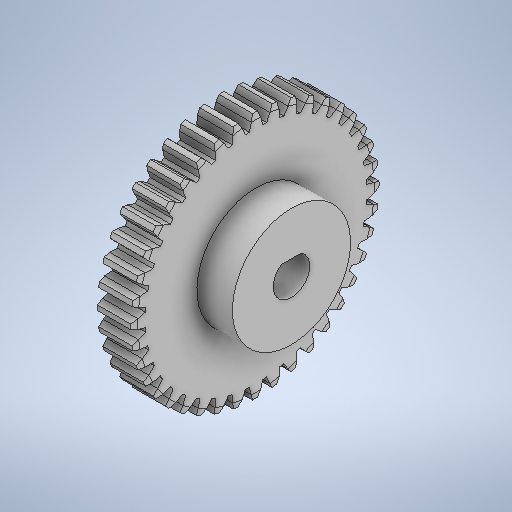
# Autodesk Inventor part: HPC - G1-40 (C)
Saved by Autodesk Inventor 2025.2 (Build 292293000, 293)
## iProperties
Category: PARTsolutions
Company: HPC
Created: 2025-05-10
Part Number: HPC - G1-40 (C)
Material: Generic
Catalog Web Link: www.cadenas.de
Description: G/PG 1-Spur gear - Steel 20NCD2 - Module 1.0
Vendor: HPC
Document SubType Name: Modeling
Designer: psAdmin
Manufacturer: HPC
Mass: 98 g
Surface Area: 56.4798 cm^2
Volume: 12.7412 cm^3
Density: 1 g/cm^3
Appearance: PSOLRGB-175-175-175
PSOL_IDENT_0: {$CADENAS_DATA/23d-libs/hpc/v4/spur_gear/100/g1.prj},171 {VTYP=3D},{NB=HPC - G1-40 (C)},{LINA=HPC -
PSOL_IDENT_1: G1-40},{NN=G/PG 1},{DATE=17.02.2022 08:08:10},{GEOMDATE=24.09.2019 07:57:00},{VERSION=},{LINEID=1130
PSOL_IDENT_2: },{WBVAR=DET},{WBNUMERIC=}  {NB=hpc_G1-40_C},{LINA=HPC - G1-40},{KT=DUMMY},{REF=G1-40},{DET=C},{TYP=
PSOL_IDENT_3: G},{MOD=1.0},{Z=40},{P=40.00},{D=42.00},{M=20},{MX=20.000},{A=8},{MAS=0.098},{INFO=INFO},{MODULE=1.0
PSOL_IDENT_4: 00},{X=37.5},{HIDDENLINE=V}
NB: HPC - G1-40 (C)
NN: G/PG 1
NT: Spur gear - Steel 20NCD2 - Module 1.0
NBSYN: HPC - $REF. ($DET.)
LINA: HPC - G1-40
CATALOG: HPC
REF: G1-40
DET: Full
TYP: G
MOD: 1.0
Z: 40
P: 40
D: 42
M: 20
A: 8
MAS: 0.098
INFO: INFO
SUPPLIER: HPC
ARTICLENO: HPC - G1-40 (C)
BOMINFO: HPC - G1-40
CREATOR: CADENAS GmbH
Title: HPC - G1-40
Author: Cadenas PARTsolutions
Comments: Spur gear - Steel 20NCD2 - Module 1.0
Autodesk Inventor part; units mm, degrees
ref_plane "YZ Plane" through (0, 0, 0) normal (1, 0, 0) x (0, 1, 0)
ref_plane "XZ Plane" through (0, 0, 0) normal (0, 1, 0) x (-1, 0, 0)
ref_plane "XY Plane" through (0, 0, 0) normal (0, 0, 1) x (1, 0, 0)
sketch "Esquisse_1" plane through (0, 0, 0) normal (0, 0, 1) x (1, 0, 0)
  line L0 (8, 0) -> (0, 0)
  line L1 (0, 20) -> (0, 0)
  line L2 (6, 20) -> (5.8237, 21)
  line L3 (5.8237, 21) -> (0.1763, 21)
  line L4 (0.1763, 21) -> (0, 20)
  line L5 (12, 0) -> (12, 10)
  line L6 (12, 10) -> (6, 10)
  line L7 (0, 0) -> (12, 0)
  line L8 (6, 10) -> (6, 20)
  dimension "d12" = 20
  dimension "d13" = 42
  dimension "d18" = 20
  dimension "d20" = 1
  dimension "d21" = 170
  dimension "d22" = 1
  dimension "d23" = 6
  dimension "d24" = 12
  constraints: 18 end point, 4 parallel, 2 horizontal, 1 vertical, 2 other
  measures "d12" diameter of L6 L0
  measures "d13" diameter of L3 L0
  measures "d18" angle of L2 L4
  measures "d20" vertical distance of L2.end L2.start
  measures "d21" angle of L4 L1
  measures "d22" vertical distance of L1.start L3.end
  measures "d23" distance between parallel lines of L8 L1
  measures "d24" distance between parallel lines of L5 L1
revolve "Revolution1" add sketch "Esquisse_1" angle 360 about axis through (8, 0, 0) along (1, 0, 0)
sketch "Esquisse_2" plane through (0, 0, 0) normal (1, 0, 0) x (0, 1, 0)
  line L0 (-23, 23) -> (-23, -23)
  line L1 (-23, -23) -> (23, -23)
  line L2 (23, -23) -> (23, 23)
  line L3 (23, 23) -> (-23, 23)
  arc A0 (0.344, 21.1972) -> (-0.344, 21.1972) centre (0, 0) ccw
  line L4 (-0.344, 21.1972) -> (-0.7854, 19.9846)
  line L5 (-0.7854, 19.9846) -> (-1.1253, 18.7162)
  arc A1 (-1.1253, 18.7162) -> (-1.8165, 18.6618) centre (0, 0) ccw
  line L6 (-1.8165, 18.6618) -> (-2.3505, 19.8614)
  line L7 (-2.3505, 19.8614) -> (-2.9762, 20.9901)
  arc A2 (-2.9762, 20.9901) -> (-3.6558, 20.8824) centre (0, 0) ccw
  line L8 (-3.6558, 20.8824) -> (-3.902, 19.6157)
  line L9 (-3.902, 19.6157) -> (-4.0393, 18.3097)
  arc A3 (-4.0393, 18.3097) -> (-4.7134, 18.1479) centre (0, 0) ccw
  line L10 (-4.7134, 18.1479) -> (-5.4286, 19.2492)
  line L11 (-5.4286, 19.2492) -> (-6.2231, 20.2661)
  arc A4 (-6.2231, 20.2661) -> (-6.8775, 20.0534) centre (0, 0) ccw
  line L12 (-6.8775, 20.0534) -> (-6.9225, 18.7638)
  line L13 (-6.9225, 18.7638) -> (-6.8538, 17.4524)
  arc A5 (-6.8538, 17.4524) -> (-7.4944, 17.1871) centre (0, 0) ccw
  line L14 (-7.4944, 17.1871) -> (-8.373, 18.1629)
  line L15 (-8.373, 18.1629) -> (-9.3168, 19.043)
  arc A6 (-9.3168, 19.043) -> (-9.9299, 18.7307) centre (0, 0) ccw
  line L16 (-9.9299, 18.7307) -> (-9.7726, 17.4498)
  line L17 (-9.7726, 17.4498) -> (-9.4996, 16.1654)
  arc A7 (-9.4996, 16.1654) -> (-10.0908, 15.8031) centre (0, 0) ccw
  line L18 (-10.0908, 15.8031) -> (-11.1112, 16.6295)
  line L19 (-11.1112, 16.6295) -> (-12.1811, 17.3511)
  arc A8 (-12.1811, 17.3511) -> (-12.7377, 16.9467) centre (0, 0) ccw
  line L20 (-12.7377, 16.9467) -> (-12.382, 15.7062)
  line L21 (-12.382, 15.7062) -> (-11.9115, 14.4803)
  arc A9 (-11.9115, 14.4803) -> (-12.4387, 14.03) centre (0, 0) ccw
  line L22 (-12.4387, 14.03) -> (-13.5759, 14.6866)
  line L23 (-13.5759, 14.6866) -> (-14.7454, 15.232)
  arc A10 (-14.7454, 15.232) -> (-15.232, 14.7454) centre (0, 0) ccw
  line L24 (-15.232, 14.7454) -> (-14.6866, 13.5759)
  line L25 (-14.6866, 13.5759) -> (-14.03, 12.4387)
  arc A11 (-14.03, 12.4387) -> (-14.4803, 11.9115) centre (0, 0) ccw
  line L26 (-14.4803, 11.9115) -> (-15.7062, 12.382)
  line L27 (-15.7062, 12.382) -> (-16.9467, 12.7377)
  arc A12 (-16.9467, 12.7377) -> (-17.3511, 12.1811) centre (0, 0) ccw
  line L28 (-17.3511, 12.1811) -> (-16.6295, 11.1112)
  line L29 (-16.6295, 11.1112) -> (-15.8031, 10.0908)
  arc A13 (-15.8031, 10.0908) -> (-16.1654, 9.4996) centre (0, 0) ccw
  line L30 (-16.1654, 9.4996) -> (-17.4498, 9.7726)
  line L31 (-17.4498, 9.7726) -> (-18.7307, 9.9299)
  arc A14 (-18.7307, 9.9299) -> (-19.043, 9.3168) centre (0, 0) ccw
  line L32 (-19.043, 9.3168) -> (-18.1629, 8.373)
  line L33 (-18.1629, 8.373) -> (-17.1871, 7.4944)
  arc A15 (-17.1871, 7.4944) -> (-17.4524, 6.8538) centre (0, 0) ccw
  line L34 (-17.4524, 6.8538) -> (-18.7638, 6.9225)
  line L35 (-18.7638, 6.9225) -> (-20.0534, 6.8775)
  arc A16 (-20.0534, 6.8775) -> (-20.2661, 6.2231) centre (0, 0) ccw
  line L36 (-20.2661, 6.2231) -> (-19.2492, 5.4286)
  line L37 (-19.2492, 5.4286) -> (-18.1479, 4.7134)
  arc A17 (-18.1479, 4.7134) -> (-18.3097, 4.0393) centre (0, 0) ccw
  line L38 (-18.3097, 4.0393) -> (-19.6157, 3.902)
  line L39 (-19.6157, 3.902) -> (-20.8824, 3.6558)
  arc A18 (-20.8824, 3.6558) -> (-20.9901, 2.9762) centre (0, 0) ccw
  line L40 (-20.9901, 2.9762) -> (-19.8614, 2.3505)
  line L41 (-19.8614, 2.3505) -> (-18.6618, 1.8165)
  arc A19 (-18.6618, 1.8165) -> (-18.7162, 1.1253) centre (0, 0) ccw
  line L42 (-18.7162, 1.1253) -> (-19.9846, 0.7854)
  line L43 (-19.9846, 0.7854) -> (-21.1972, 0.344)
  arc A20 (-21.1972, 0.344) -> (-21.1972, -0.344) centre (0, 0) ccw
  line L44 (-21.1972, -0.344) -> (-19.9846, -0.7854)
  line L45 (-19.9846, -0.7854) -> (-18.7162, -1.1253)
  arc A21 (-18.7162, -1.1253) -> (-18.6618, -1.8165) centre (0, 0) ccw
  line L46 (-18.6618, -1.8165) -> (-19.8614, -2.3505)
  line L47 (-19.8614, -2.3505) -> (-20.9901, -2.9762)
  arc A22 (-20.9901, -2.9762) -> (-20.8824, -3.6558) centre (0, 0) ccw
  line L48 (-20.8824, -3.6558) -> (-19.6157, -3.902)
  line L49 (-19.6157, -3.902) -> (-18.3097, -4.0393)
  arc A23 (-18.3097, -4.0393) -> (-18.1479, -4.7134) centre (0, 0) ccw
  line L50 (-18.1479, -4.7134) -> (-19.2492, -5.4286)
  line L51 (-19.2492, -5.4286) -> (-20.2661, -6.2231)
  arc A24 (-20.2661, -6.2231) -> (-20.0534, -6.8775) centre (0, 0) ccw
  line L52 (-20.0534, -6.8775) -> (-18.7638, -6.9225)
  line L53 (-18.7638, -6.9225) -> (-17.4524, -6.8538)
  arc A25 (-17.4524, -6.8538) -> (-17.1871, -7.4944) centre (0, 0) ccw
  line L54 (-17.1871, -7.4944) -> (-18.1629, -8.373)
  line L55 (-18.1629, -8.373) -> (-19.043, -9.3168)
  arc A26 (-19.043, -9.3168) -> (-18.7307, -9.9299) centre (0, 0) ccw
  line L56 (-18.7307, -9.9299) -> (-17.4498, -9.7726)
  line L57 (-17.4498, -9.7726) -> (-16.1654, -9.4996)
  arc A27 (-16.1654, -9.4996) -> (-15.8031, -10.0908) centre (0, 0) ccw
  line L58 (-15.8031, -10.0908) -> (-16.6295, -11.1112)
  line L59 (-16.6295, -11.1112) -> (-17.3511, -12.1811)
  arc A28 (-17.3511, -12.1811) -> (-16.9467, -12.7377) centre (0, 0) ccw
  line L60 (-16.9467, -12.7377) -> (-15.7062, -12.382)
  line L61 (-15.7062, -12.382) -> (-14.4803, -11.9115)
  arc A29 (-14.4803, -11.9115) -> (-14.03, -12.4387) centre (0, 0) ccw
  line L62 (-14.03, -12.4387) -> (-14.6866, -13.5759)
  line L63 (-14.6866, -13.5759) -> (-15.232, -14.7454)
  arc A30 (-15.232, -14.7454) -> (-14.7454, -15.232) centre (0, 0) ccw
  line L64 (-14.7454, -15.232) -> (-13.5759, -14.6866)
  line L65 (-13.5759, -14.6866) -> (-12.4387, -14.03)
  arc A31 (-12.4387, -14.03) -> (-11.9115, -14.4803) centre (0, 0) ccw
  line L66 (-11.9115, -14.4803) -> (-12.382, -15.7062)
  line L67 (-12.382, -15.7062) -> (-12.7377, -16.9467)
  arc A32 (-12.7377, -16.9467) -> (-12.1811, -17.3511) centre (0, 0) ccw
  line L68 (-12.1811, -17.3511) -> (-11.1112, -16.6295)
  line L69 (-11.1112, -16.6295) -> (-10.0908, -15.8031)
  arc A33 (-10.0908, -15.8031) -> (-9.4996, -16.1654) centre (0, 0) ccw
  line L70 (-9.4996, -16.1654) -> (-9.7726, -17.4498)
  line L71 (-9.7726, -17.4498) -> (-9.9299, -18.7307)
  arc A34 (-9.9299, -18.7307) -> (-9.3168, -19.043) centre (0, 0) ccw
  line L72 (-9.3168, -19.043) -> (-8.373, -18.1629)
  line L73 (-8.373, -18.1629) -> (-7.4944, -17.1871)
  arc A35 (-7.4944, -17.1871) -> (-6.8538, -17.4524) centre (0, 0) ccw
  line L74 (-6.8538, -17.4524) -> (-6.9225, -18.7638)
  line L75 (-6.9225, -18.7638) -> (-6.8775, -20.0534)
  arc A36 (-6.8775, -20.0534) -> (-6.2231, -20.2661) centre (0, 0) ccw
  line L76 (-6.2231, -20.2661) -> (-5.4286, -19.2492)
  line L77 (-5.4286, -19.2492) -> (-4.7134, -18.1479)
  arc A37 (-4.7134, -18.1479) -> (-4.0393, -18.3097) centre (0, 0) ccw
  line L78 (-4.0393, -18.3097) -> (-3.902, -19.6157)
  line L79 (-3.902, -19.6157) -> (-3.6558, -20.8824)
  arc A38 (-3.6558, -20.8824) -> (-2.9762, -20.9901) centre (0, 0) ccw
  line L80 (-2.9762, -20.9901) -> (-2.3505, -19.8614)
  line L81 (-2.3505, -19.8614) -> (-1.8165, -18.6618)
  arc A39 (-1.8165, -18.6618) -> (-1.1253, -18.7162) centre (0, 0) ccw
  line L82 (-1.1253, -18.7162) -> (-0.7854, -19.9846)
  line L83 (-0.7854, -19.9846) -> (-0.344, -21.1972)
  arc A40 (-0.344, -21.1972) -> (0.344, -21.1972) centre (0, 0) ccw
  line L84 (0.344, -21.1972) -> (0.7854, -19.9846)
  line L85 (0.7854, -19.9846) -> (1.1253, -18.7162)
  arc A41 (1.1253, -18.7162) -> (1.8165, -18.6618) centre (0, 0) ccw
  line L86 (1.8165, -18.6618) -> (2.3505, -19.8614)
  line L87 (2.3505, -19.8614) -> (2.9762, -20.9901)
  arc A42 (2.9762, -20.9901) -> (3.6558, -20.8824) centre (0, 0) ccw
  line L88 (3.6558, -20.8824) -> (3.902, -19.6157)
  line L89 (3.902, -19.6157) -> (4.0393, -18.3097)
  arc A43 (4.0393, -18.3097) -> (4.7134, -18.1479) centre (0, 0) ccw
  line L90 (4.7134, -18.1479) -> (5.4286, -19.2492)
  line L91 (5.4286, -19.2492) -> (6.2231, -20.2661)
  arc A44 (6.2231, -20.2661) -> (6.8775, -20.0534) centre (0, 0) ccw
  line L92 (6.8775, -20.0534) -> (6.9225, -18.7638)
  line L93 (6.9225, -18.7638) -> (6.8538, -17.4524)
  arc A45 (6.8538, -17.4524) -> (7.4944, -17.1871) centre (0, 0) ccw
  line L94 (7.4944, -17.1871) -> (8.373, -18.1629)
  line L95 (8.373, -18.1629) -> (9.3168, -19.043)
  arc A46 (9.3168, -19.043) -> (9.9299, -18.7307) centre (0, 0) ccw
  line L96 (9.9299, -18.7307) -> (9.7726, -17.4498)
  line L97 (9.7726, -17.4498) -> (9.4996, -16.1654)
  arc A47 (9.4996, -16.1654) -> (10.0908, -15.8031) centre (0, 0) ccw
  line L98 (10.0908, -15.8031) -> (11.1112, -16.6295)
  line L99 (11.1112, -16.6295) -> (12.1811, -17.3511)
  arc A48 (12.1811, -17.3511) -> (12.7377, -16.9467) centre (0, 0) ccw
  line L100 (12.7377, -16.9467) -> (12.382, -15.7062)
  line L101 (12.382, -15.7062) -> (11.9115, -14.4803)
  arc A49 (11.9115, -14.4803) -> (12.4387, -14.03) centre (0, 0) ccw
  line L102 (12.4387, -14.03) -> (13.5759, -14.6866)
  line L103 (13.5759, -14.6866) -> (14.7454, -15.232)
  arc A50 (14.7454, -15.232) -> (15.232, -14.7454) centre (0, 0) ccw
  line L104 (15.232, -14.7454) -> (14.6866, -13.5759)
  line L105 (14.6866, -13.5759) -> (14.03, -12.4387)
  arc A51 (14.03, -12.4387) -> (14.4803, -11.9115) centre (0, 0) ccw
  line L106 (14.4803, -11.9115) -> (15.7062, -12.382)
  line L107 (15.7062, -12.382) -> (16.9467, -12.7377)
  arc A52 (16.9467, -12.7377) -> (17.3511, -12.1811) centre (0, 0) ccw
  line L108 (17.3511, -12.1811) -> (16.6295, -11.1112)
  line L109 (16.6295, -11.1112) -> (15.8031, -10.0908)
  arc A53 (15.8031, -10.0908) -> (16.1654, -9.4996) centre (0, 0) ccw
  line L110 (16.1654, -9.4996) -> (17.4498, -9.7726)
  line L111 (17.4498, -9.7726) -> (18.7307, -9.9299)
  arc A54 (18.7307, -9.9299) -> (19.043, -9.3168) centre (0, 0) ccw
  line L112 (19.043, -9.3168) -> (18.1629, -8.373)
  line L113 (18.1629, -8.373) -> (17.1871, -7.4944)
  arc A55 (17.1871, -7.4944) -> (17.4524, -6.8538) centre (0, 0) ccw
  line L114 (17.4524, -6.8538) -> (18.7638, -6.9225)
  line L115 (18.7638, -6.9225) -> (20.0534, -6.8775)
  arc A56 (20.0534, -6.8775) -> (20.2661, -6.2231) centre (0, 0) ccw
  line L116 (20.2661, -6.2231) -> (19.2492, -5.4286)
  line L117 (19.2492, -5.4286) -> (18.1479, -4.7134)
  arc A57 (18.1479, -4.7134) -> (18.3097, -4.0393) centre (0, 0) ccw
  line L118 (18.3097, -4.0393) -> (19.6157, -3.902)
  line L119 (19.6157, -3.902) -> (20.8824, -3.6558)
  arc A58 (20.8824, -3.6558) -> (20.9901, -2.9762) centre (0, 0) ccw
  line L120 (20.9901, -2.9762) -> (19.8614, -2.3505)
  line L121 (19.8614, -2.3505) -> (18.6618, -1.8165)
  arc A59 (18.6618, -1.8165) -> (18.7162, -1.1253) centre (0, 0) ccw
  line L122 (18.7162, -1.1253) -> (19.9846, -0.7854)
  line L123 (19.9846, -0.7854) -> (21.1972, -0.344)
  arc A60 (21.1972, -0.344) -> (21.1972, 0.344) centre (0, 0) ccw
  line L124 (21.1972, 0.344) -> (19.9846, 0.7854)
  line L125 (19.9846, 0.7854) -> (18.7162, 1.1253)
  arc A61 (18.7162, 1.1253) -> (18.6618, 1.8165) centre (0, 0) ccw
  line L126 (18.6618, 1.8165) -> (19.8614, 2.3505)
  line L127 (19.8614, 2.3505) -> (20.9901, 2.9762)
  arc A62 (20.9901, 2.9762) -> (20.8824, 3.6558) centre (0, 0) ccw
  line L128 (20.8824, 3.6558) -> (19.6157, 3.902)
  line L129 (19.6157, 3.902) -> (18.3097, 4.0393)
  arc A63 (18.3097, 4.0393) -> (18.1479, 4.7134) centre (0, 0) ccw
  line L130 (18.1479, 4.7134) -> (19.2492, 5.4286)
  line L131 (19.2492, 5.4286) -> (20.2661, 6.2231)
  arc A64 (20.2661, 6.2231) -> (20.0534, 6.8775) centre (0, 0) ccw
  line L132 (20.0534, 6.8775) -> (18.7638, 6.9225)
  line L133 (18.7638, 6.9225) -> (17.4524, 6.8538)
  arc A65 (17.4524, 6.8538) -> (17.1871, 7.4944) centre (0, 0) ccw
  line L134 (17.1871, 7.4944) -> (18.1629, 8.373)
  line L135 (18.1629, 8.373) -> (19.043, 9.3168)
  arc A66 (19.043, 9.3168) -> (18.7307, 9.9299) centre (0, 0) ccw
  line L136 (18.7307, 9.9299) -> (17.4498, 9.7726)
  line L137 (17.4498, 9.7726) -> (16.1654, 9.4996)
  arc A67 (16.1654, 9.4996) -> (15.8031, 10.0908) centre (0, 0) ccw
  line L138 (15.8031, 10.0908) -> (16.6295, 11.1112)
  line L139 (16.6295, 11.1112) -> (17.3511, 12.1811)
  arc A68 (17.3511, 12.1811) -> (16.9467, 12.7377) centre (0, 0) ccw
  line L140 (16.9467, 12.7377) -> (15.7062, 12.382)
  line L141 (15.7062, 12.382) -> (14.4803, 11.9115)
  arc A69 (14.4803, 11.9115) -> (14.03, 12.4387) centre (0, 0) ccw
  line L142 (14.03, 12.4387) -> (14.6866, 13.5759)
  line L143 (14.6866, 13.5759) -> (15.232, 14.7454)
  arc A70 (15.232, 14.7454) -> (14.7454, 15.232) centre (0, 0) ccw
  line L144 (14.7454, 15.232) -> (13.5759, 14.6866)
  line L145 (13.5759, 14.6866) -> (12.4387, 14.03)
  arc A71 (12.4387, 14.03) -> (11.9115, 14.4803) centre (0, 0) ccw
  line L146 (11.9115, 14.4803) -> (12.382, 15.7062)
  line L147 (12.382, 15.7062) -> (12.7377, 16.9467)
  arc A72 (12.7377, 16.9467) -> (12.1811, 17.3511) centre (0, 0) ccw
  line L148 (12.1811, 17.3511) -> (11.1112, 16.6295)
  line L149 (11.1112, 16.6295) -> (10.0908, 15.8031)
  arc A73 (10.0908, 15.8031) -> (9.4996, 16.1654) centre (0, 0) ccw
  line L150 (9.4996, 16.1654) -> (9.7726, 17.4498)
  line L151 (9.7726, 17.4498) -> (9.9299, 18.7307)
  arc A74 (9.9299, 18.7307) -> (9.3168, 19.043) centre (0, 0) ccw
  line L152 (9.3168, 19.043) -> (8.373, 18.1629)
  line L153 (8.373, 18.1629) -> (7.4944, 17.1871)
  arc A75 (7.4944, 17.1871) -> (6.8538, 17.4524) centre (0, 0) ccw
  line L154 (6.8538, 17.4524) -> (6.9225, 18.7638)
  line L155 (6.9225, 18.7638) -> (6.8775, 20.0534)
  arc A76 (6.8775, 20.0534) -> (6.2231, 20.2661) centre (0, 0) ccw
  line L156 (6.2231, 20.2661) -> (5.4286, 19.2492)
  line L157 (5.4286, 19.2492) -> (4.7134, 18.1479)
  arc A77 (4.7134, 18.1479) -> (4.0393, 18.3097) centre (0, 0) ccw
  line L158 (4.0393, 18.3097) -> (3.902, 19.6157)
  line L159 (3.902, 19.6157) -> (3.6558, 20.8824)
  arc A78 (3.6558, 20.8824) -> (2.9762, 20.9901) centre (0, 0) ccw
  line L160 (2.9762, 20.9901) -> (2.3505, 19.8614)
  line L161 (2.3505, 19.8614) -> (1.8165, 18.6618)
  arc A79 (1.8165, 18.6618) -> (1.1253, 18.7162) centre (0, 0) ccw
  line L162 (1.1253, 18.7162) -> (0.7854, 19.9846)
  line L163 (0.7854, 19.9846) -> (0.344, 21.1972)
  constraints: 328 end point, 160 point on circle, 80 centre point
extrude "Extrusion1" cut sketch "Esquisse_2" along normal blind 8
sketch "Esquisse7" plane through (12, 0, 0) normal (1, 0, 0) x (0, 0, -1)
  arc A0 (-1.6882, 2.6) -> (1.6882, 2.6) centre (0, 0) ccw
  line L0 (-1.6882, 2.6) -> (1.6882, 2.6)
  dimension "d25" = 6.2
  dimension "d26" = 2.6
  constraints: 2 end point, 2 point on circle, 1 centre point, 1 coincident, 1 horizontal
  measures "d25" diameter of A0
  measures "d26" distance from line of point (0, 0) L0
extrude "Extrusion5" cut sketch "Esquisse7" against normal through all
body "Solid1"
